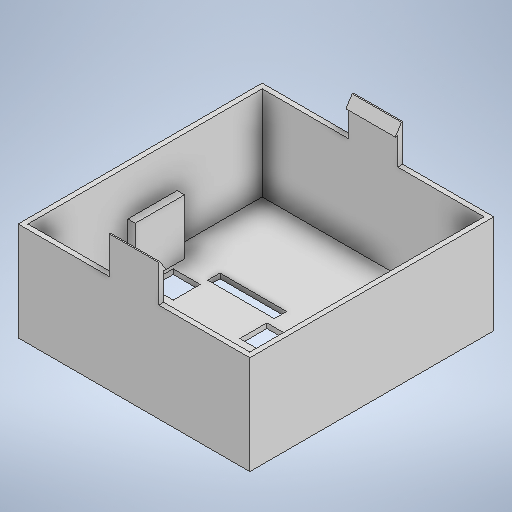
# Autodesk Inventor part: Arduino_case_lid
Saved by Autodesk Inventor 2025.2 (Build 292293000, 293)
## iProperties
Created: 2025-09-19
Part Number: Arduino_case_lid
Material: Generic
Document SubType Name: Modeling
Designer: TSO
Density: 1 g/cm^3
Appearance: Default
Author: TSO
Autodesk Inventor part; units mm, degrees
ref_plane "YZ Plane" through (0, 0, 0) normal (1, 0, 0) x (0, 1, 0)
ref_plane "XZ Plane" through (0, 0, 0) normal (0, 1, 0) x (-1, 0, 0)
ref_plane "XY Plane" through (0, 0, 0) normal (0, 0, 1) x (1, 0, 0)
sketch "Sketch1" plane through (0, 0, 0) normal (0, 1, 0) x (-1, 0, 0)
  line L0 (0, 0) -> (94, 0)
  line L1 (94, 0) -> (94, -99)
  line L2 (94, -99) -> (0, -99)
  line L3 (0, -99) -> (0, 0)
  dimension "d0" = 94
  dimension "d1" = 99
  constraints: 8 end point, 2 parallel, 1 horizontal, 1 perpendicular
  measures "d0" distance of L1.end L2.end
  measures "d1" distance of L0.end L1.end
extrude "Extrusion1" add sketch "Sketch1" along normal blind 40
sketch "Sketch2" plane through (0, 40, 0) normal (0, 1, 0) x (1, 0, 0)
  line L0 (0, 0) -> (0, 99) projected
  line L1 (0, 0) -> (-2, 0)
  line L2 (-2, 0) -> (-2, 2)
  line L3 (-2, 2) -> (0, 2)
  line L4 (0, 2) -> (0, 0)
  line L5 (-2, 2) -> (-92, 2)
  line L6 (-92, 2) -> (-92, 97)
  line L7 (-92, 97) -> (-2, 97)
  line L8 (-2, 97) -> (-2, 2)
  dimension "d4" = 2
  dimension "d5" = 2
  dimension "d6" = 90
  dimension "d7" = 95
  constraints: 16 end point, 4 parallel, 2 horizontal, 2 perpendicular
  measures "d4" distance of L2.end L3.end
  measures "d5" distance of L1.end L2.end
  measures "d6" distance of L6.end L7.end
  measures "d7" distance of L5.end L6.end
extrude "Extrusion2" cut sketch "Sketch2" against normal blind 38 contours L5 L6 L7 L8
sketch "Sketch3" plane through (0, 40, 0) normal (0, 1, 0) x (1, 0, 0)
  line L0 (-92, 97) -> (-2, 97) projected
  line L1 (0, 99) -> (-94, 99) projected
  line L2 (-92, 2) -> (-92, 97) projected
  line L3 (-92, 97) -> (-57, 97)
  line L4 (-92, 97) -> (-57, 97) construction
  line L5 (-57, 97) -> (-37, 97)
  line L6 (-37, 97) -> (-37, 99)
  line L7 (-37, 99) -> (-57, 99)
  line L8 (-57, 99) -> (-57, 97)
  line L9 (-2, 2) -> (-92, 2) projected
  line L10 (-94, 0) -> (0, 0) projected
  line L11 (-57, 2) -> (-37, 2)
  line L12 (-37, 2) -> (-37, 0)
  line L13 (-37, 0) -> (-57, 0)
  line L14 (-57, 0) -> (-57, 2)
  dimension "d11" = 35
  dimension "d12" = 0
  dimension "d13" = 20
  dimension "d14" = 20
  constraints: 20 end point, 4 parallel, 3 horizontal, 3 point on line, 2 collinear, 2 perpendicular
  measures "d11" distance of L0.start L3.end
  measures "d12" distance between parallel lines of L4 L3
  measures "d13" distance of L7.end L6.end
  measures "d14" distance of L12.end L13.end
extrude "Extrusion3" add sketch "Sketch3" along normal blind 15
sketch "Sketch4" plane through (-92, 2, -97) normal (0, 0, 1) x (1, 0, 0)
  line L0 (35, 38) -> (35, 53) projected
  line L1 (35, 53) -> (55, 53)
  line L2 (55, 53) -> (55, 49)
  line L3 (55, 49) -> (35, 49)
  line L4 (35, 49) -> (35, 53)
  point P0 (92, -2)
  dimension "d17" = 20
  dimension "d18" = 4
  constraints: 8 end point, 2 parallel, 1 horizontal, 1 perpendicular
  measures "d17" distance of L2.end L3.end
  measures "d18" distance of L1.end L2.end
extrude "Extrusion4" add sketch "Sketch4" along normal up to surface (95 mm away)
sketch "Sketch5" plane through (0, 55, 0) normal (0, 1, 0) x (1, 0, 0)
  line L0 (-57, 2) -> (-92, 2) projected
  line L1 (-57, 2) -> (-57, 3)
  line L2 (-57, 97) -> (-57, 2) projected
  line L3 (-57, 3) -> (-37, 3)
  line L4 (-37, 3) -> (-37, 96)
  line L5 (-37, 96) -> (-57, 96)
  line L6 (-57, 96) -> (-57, 3)
  point P0 (0, 0)
  dimension "d21" = 1
  dimension "d22" = 93
  constraints: 10 end point, 2 parallel, 1 horizontal, 1 perpendicular, 1 point on line
  measures "d21" distance of L0.start L1.end
  measures "d22" distance of L4.end L3.end
extrude "Extrusion5" cut sketch "Sketch5" against normal up to surface (4 mm away)
chamfer "Chamfer1" distance 2.5 distance2 4 1 edges at (-47, 55, -96) measured on face at (-50.3333, 55, -98)
chamfer "Chamfer2" distance 2.5 distance2 4 1 edges at (-47, 55, -3) measured on face at (-50.3333, 55, -1)
sketch "Sketch6" plane through (0, 2, 0) normal (0, 1, 0) x (1, 0, 0)
  line L0 (-92, 2) -> (-92, 97) projected
  line L1 (-92, 2) -> (-89, 2)
  line L2 (-89, 2) -> (-89, 5) construction
  line L3 (-89, 5) -> (-92, 5) construction
  line L4 (-92, 5) -> (-92, 2)
  line L5 (-89, 5) -> (-89, 39.5) construction
  line L6 (-92, 97) -> (-57, 97) projected
  line L7 (-89, 39.5) -> (-86, 39.5)
  line L8 (-86, 39.5) -> (-86, 59.5)
  line L9 (-86, 59.5) -> (-89, 59.5)
  line L10 (-89, 59.5) -> (-89, 39.5)
  line L11 (0, 99) -> (-94, 99) projected
  line L12 (-47, 99) -> (-47, 0) construction
  line L13 (-94, 0) -> (0, 0) projected
  line L14 (-5, 39.5) -> (-8, 39.5)
  line L15 (-8, 39.5) -> (-8, 59.5)
  line L16 (-8, 59.5) -> (-5, 59.5)
  line L17 (-5, 59.5) -> (-5, 39.5)
  dimension "d31" = 3
  dimension "d32" = 3
  dimension "d33" = 34.5
  dimension "d34" = 3
  dimension "d35" = 20
  dimension "d36" = 37.5
  constraints: 28 end point, 4 parallel, 4 symmetric about line, 3 perpendicular, 2 horizontal, 2 midpoint
  measures "d31" distance of L3.end L2.end
  measures "d32" distance of L2.end L1.end
  measures "d33" distance of L2.end L5.end
  measures "d34" distance of L9.end L8.end
  measures "d35" distance of L8.end L7.end
  measures "d36" distance from line of L6 L9.end
extrude "Extrusion6" add sketch "Sketch6" along normal blind 22.5
sketch "Sketch7" plane through (0, 0, 0) normal (0, -1, 0) x (1, 0, 0)
  line L0 (-94, 0) -> (0, 0) projected
  line L1 (-94, 0) -> (-90, 0)
  line L2 (-90, 0) -> (-90, -4) construction
  line L3 (-90, -4) -> (-94, -4) construction
  line L4 (-94, -4) -> (-94, 0)
  line L5 (-90, -4) -> (-84.8, -4) construction
  line L6 (-84.8, -4) -> (-84.8, -42.7) construction
  line L7 (-84.8, -42.7) -> (-90, -42.7) construction
  line L8 (-90, -42.7) -> (-90, -4) construction
  line L9 (-84.8, -42.7) -> (-73.8, -42.7)
  line L10 (-73.8, -42.7) -> (-73.8, -53.7)
  line L11 (-73.8, -53.7) -> (-84.8, -53.7)
  line L12 (-84.8, -53.7) -> (-84.8, -42.7)
  line L13 (-73.8, -53.7) -> (-46.8, -53.7) construction
  line L14 (-46.8, -53.7) -> (-46.8, -56.7) construction
  line L15 (-46.8, -56.7) -> (-73.8, -56.7) construction
  line L16 (-73.8, -56.7) -> (-73.8, -53.7) construction
  line L17 (-46.8, -56.7) -> (-73.8, -56.7)
  line L18 (-73.8, -56.7) -> (-73.8, -61.7)
  line L19 (-73.8, -61.7) -> (-46.8, -61.7)
  line L20 (-46.8, -61.7) -> (-46.8, -56.7)
  line L21 (-46.8, -53.7) -> (-35.8, -53.7)
  line L22 (-35.8, -53.7) -> (-35.8, -42.7)
  line L23 (-35.8, -42.7) -> (-46.8, -42.7)
  line L24 (-46.8, -42.7) -> (-46.8, -53.7)
  dimension "d39" = 4
  dimension "d40" = 4
  dimension "d41" = 5.2
  dimension "d42" = 38.7
  dimension "d43" = 11
  dimension "d44" = 11
  dimension "d45" = 27
  dimension "d46" = 3
  dimension "d47" = 5
  dimension "d48" = 11
  dimension "d49" = 11
  constraints: 48 end point, 12 parallel, 6 horizontal, 6 perpendicular
  measures "d39" distance of L2.end L3.end
  measures "d40" distance of L1.end L2.end
  measures "d41" distance of L6.end L7.end
  measures "d42" distance of L5.end L6.end
  measures "d43" distance of L10.end L11.end
  measures "d44" distance of L9.end L10.end
  measures "d45" distance of L14.end L15.end
  measures "d46" distance of L13.end L14.end
  measures "d47" distance of L18.end L17.end
  measures "d48" distance of L23.end L22.end
  measures "d49" distance of L22.end L21.end
extrude "Extrusion7" cut sketch "Sketch7" against normal up to surface (2 mm away)
sketch "Sketch8" plane through (0, 0, 0) normal (0, -1, 0) x (1, 0, 0)
  line L0 (0, -99) -> (-94, -99) projected
  line L1 (0, -99) -> (-23.5, -99)
  line L2 (-23.5, -99) -> (-23.5, -89.75)
  line L3 (-23.5, -89.75) -> (0, -89.75)
  line L4 (0, -89.75) -> (0, -99)
  line L5 (-23.5, -89.75) -> (-70.5, -89.75)
  line L6 (-70.5, -89.75) -> (-70.5, -71.25)
  line L7 (-70.5, -71.25) -> (-23.5, -71.25)
  line L8 (-23.5, -71.25) -> (-23.5, -89.75)
  line L9 (-23.3088, -89.836) -> (-70.529, -89.836) construction
  line L10 (-70.529, -89.836) -> (-70.529, -70.9161) construction
  line L11 (-70.529, -70.9161) -> (-23.3088, -70.9161) construction
  line L12 (-23.3088, -70.9161) -> (-23.3088, -89.836) construction
  line L13 (0, -99) -> (-47, -99)
  line L14 (-47, -99) -> (-47, -80.5) construction
  line L15 (-47, -80.5) -> (0, -80.5) construction
  line L16 (0, -80.5) -> (0, -99)
  line L17 (-23.29, -78.926) -> (-24.2676, -81.826)
  line L18 (-24.2676, -81.826) -> (-24.7423, -81.826)
  line L19 (-24.7423, -81.826) -> (-25.72, -78.926)
  line L20 (-25.72, -78.926) -> (-25.3134, -78.926)
  line L21 (-25.3134, -78.926) -> (-25.0502, -79.7368)
  line L22 (-25.0502, -79.7368) -> (-23.9433, -79.7368)
  line L23 (-23.9433, -79.7368) -> (-23.6801, -78.926)
  line L24 (-23.6801, -78.926) -> (-23.29, -78.926)
  line L25 (-24.9444, -80.0658) -> (-24.4956, -81.4312)
  line L26 (-24.4956, -81.4312) -> (-24.0491, -80.0658)
  line L27 (-24.0491, -80.0658) -> (-24.9444, -80.0658)
  line L28 (-27.0055, -78.926) -> (-25.8821, -78.926)
  line L29 (-25.8821, -78.926) -> (-25.8821, -79.2222)
  line L30 (-25.8821, -79.2222) -> (-26.2511, -79.2222)
  line L31 (-26.2511, -79.2222) -> (-26.2511, -81.5299)
  line L32 (-26.2511, -81.5299) -> (-25.8821, -81.5299)
  line L33 (-25.8821, -81.5299) -> (-25.8821, -81.826)
  line L34 (-25.8821, -81.826) -> (-27.0055, -81.826)
  line L35 (-27.0055, -81.826) -> (-27.0055, -81.5299)
  line L36 (-27.0055, -81.5299) -> (-26.6365, -81.5299)
  line L37 (-26.6365, -81.5299) -> (-26.6365, -79.2222)
  line L38 (-26.6365, -79.2222) -> (-27.0055, -79.2222)
  line L39 (-27.0055, -79.2222) -> (-27.0055, -78.926)
  line L40 (-29.7269, -78.926) -> (-29.2263, -78.926)
  line L41 (-29.2263, -78.926) -> (-28.3098, -80.0799)
  line L42 (-28.3098, -80.0799) -> (-27.8679, -80.0799)
  line L43 (-27.8679, -80.0799) -> (-27.8679, -78.926)
  line L44 (-27.8679, -78.926) -> (-27.4825, -78.926)
  line L45 (-27.4825, -78.926) -> (-27.4825, -81.826)
  line L46 (-27.4825, -81.826) -> (-28.2299, -81.826)
  spline S0 degree 2 poles (-28.2299, -81.826) (-28.479, -81.826) (-28.815, -81.772) (-28.9678, -81.6733) knots 0 0 0 1 2 2 2
  spline S1 degree 2 poles (-28.9678, -81.6733) (-29.1205, -81.5746) (-29.2968, -81.2667) (-29.2968, -81.0388) knots 0 0 0 1 2 2 2
  spline S2 degree 2 poles (-29.2968, -81.0388) (-29.2968, -80.7215) (-28.9725, -80.2914) (-28.6952, -80.188) knots 0 0 0 1 2 2 2
  line L47 (-28.6952, -80.188) -> (-29.7269, -78.926)
  spline S3 degree 2 poles (-28.8949, -81.0082) (-28.8949, -81.1351) (-28.8056, -81.3302) (-28.7116, -81.3936) knots 0 0 0 1 2 2 2
  spline S4 degree 2 poles (-28.7116, -81.3936) (-28.6294, -81.4477) (-28.4108, -81.4923) (-28.251, -81.4923) knots 0 0 0 1 2 2 2
  line L48 (-28.251, -81.4923) -> (-27.8679, -81.4923)
  line L49 (-27.8679, -81.4923) -> (-27.8679, -80.4019)
  line L50 (-27.8679, -80.4019) -> (-28.2064, -80.4019)
  spline S5 degree 2 poles (-28.2064, -80.4019) (-28.3732, -80.4019) (-28.6388, -80.4606) (-28.7304, -80.5523) knots 0 0 0 1 2 2 2
  spline S6 degree 2 poles (-28.7304, -80.5523) (-28.815, -80.6322) (-28.8949, -80.8578) (-28.8949, -81.0082) knots 0 0 0 1 2 2 2
  line L51 (-33.3084, -78.926) -> (-32.923, -78.926)
  line L52 (-32.923, -78.926) -> (-32.923, -80.3455)
  line L53 (-32.923, -80.3455) -> (-31.5881, -80.3455)
  line L54 (-31.5881, -80.3455) -> (-31.5881, -78.926)
  line L55 (-31.5881, -78.926) -> (-31.2027, -78.926)
  line L56 (-31.2027, -78.926) -> (-31.2027, -81.826)
  line L57 (-31.2027, -81.826) -> (-31.5881, -81.826)
  line L58 (-31.5881, -81.826) -> (-31.5881, -80.6886)
  line L59 (-31.5881, -80.6886) -> (-32.923, -80.6886)
  line L60 (-32.923, -80.6886) -> (-32.923, -81.826)
  line L61 (-32.923, -81.826) -> (-33.3084, -81.826)
  line L62 (-33.3084, -81.826) -> (-33.3084, -78.926)
  line L63 (-33.8959, -78.926) -> (-33.8959, -81.826)
  line L64 (-33.8959, -81.826) -> (-35.7102, -81.826)
  line L65 (-35.7102, -81.826) -> (-35.7102, -81.4829)
  line L66 (-35.7102, -81.4829) -> (-34.2813, -81.4829)
  line L67 (-34.2813, -81.4829) -> (-34.2813, -80.6886)
  line L68 (-34.2813, -80.6886) -> (-35.6138, -80.6886)
  line L69 (-35.6138, -80.6886) -> (-35.6138, -80.3455)
  line L70 (-35.6138, -80.3455) -> (-34.2813, -80.3455)
  line L71 (-34.2813, -80.3455) -> (-34.2813, -79.2692)
  line L72 (-34.2813, -79.2692) -> (-35.7102, -79.2692)
  line L73 (-35.7102, -79.2692) -> (-35.7102, -78.926)
  line L74 (-35.7102, -78.926) -> (-33.8959, -78.926)
  line L75 (-35.8206, -78.926) -> (-36.7983, -81.826)
  line L76 (-36.7983, -81.826) -> (-37.273, -81.826)
  line L77 (-37.273, -81.826) -> (-38.2506, -78.926)
  line L78 (-38.2506, -78.926) -> (-37.844, -78.926)
  line L79 (-37.844, -78.926) -> (-37.5808, -79.7368)
  line L80 (-37.5808, -79.7368) -> (-36.4739, -79.7368)
  line L81 (-36.4739, -79.7368) -> (-36.2107, -78.926)
  line L82 (-36.2107, -78.926) -> (-35.8206, -78.926)
  line L83 (-37.4751, -80.0658) -> (-37.0262, -81.4312)
  line L84 (-37.0262, -81.4312) -> (-36.5797, -80.0658)
  line L85 (-36.5797, -80.0658) -> (-37.4751, -80.0658)
  line L86 (-39.2024, -78.926) -> (-39.2024, -81.4829)
  line L87 (-39.2024, -81.4829) -> (-38.2295, -81.4829)
  line L88 (-38.2295, -81.4829) -> (-38.2295, -81.826)
  line L89 (-38.2295, -81.826) -> (-40.5607, -81.826)
  line L90 (-40.5607, -81.826) -> (-40.5607, -81.4829)
  line L91 (-40.5607, -81.4829) -> (-39.5878, -81.4829)
  line L92 (-39.5878, -81.4829) -> (-39.5878, -78.926)
  line L93 (-39.5878, -78.926) -> (-39.2024, -78.926)
  line L94 (-40.8545, -78.926) -> (-40.8545, -81.826)
  line L95 (-40.8545, -81.826) -> (-42.6688, -81.826)
  line L96 (-42.6688, -81.826) -> (-42.6688, -81.4829)
  line L97 (-42.6688, -81.4829) -> (-41.2399, -81.4829)
  line L98 (-41.2399, -81.4829) -> (-41.2399, -80.6886)
  line L99 (-41.2399, -80.6886) -> (-42.5724, -80.6886)
  line L100 (-42.5724, -80.6886) -> (-42.5724, -80.3455)
  line L101 (-42.5724, -80.3455) -> (-41.2399, -80.3455)
  line L102 (-41.2399, -80.3455) -> (-41.2399, -79.2692)
  line L103 (-41.2399, -79.2692) -> (-42.6688, -79.2692)
  line L104 (-42.6688, -79.2692) -> (-42.6688, -78.926)
  line L105 (-42.6688, -78.926) -> (-40.8545, -78.926)
  line L106 (-45.3361, -78.926) -> (-44.8355, -78.926)
  line L107 (-44.8355, -78.926) -> (-43.919, -80.0799)
  line L108 (-43.919, -80.0799) -> (-43.4772, -80.0799)
  line L109 (-43.4772, -80.0799) -> (-43.4772, -78.926)
  line L110 (-43.4772, -78.926) -> (-43.0918, -78.926)
  line L111 (-43.0918, -78.926) -> (-43.0918, -81.826)
  line L112 (-43.0918, -81.826) -> (-43.8391, -81.826)
  spline S7 degree 2 poles (-43.8391, -81.826) (-44.0882, -81.826) (-44.4243, -81.772) (-44.577, -81.6733) knots 0 0 0 1 2 2 2
  spline S8 degree 2 poles (-44.577, -81.6733) (-44.7298, -81.5746) (-44.906, -81.2667) (-44.906, -81.0388) knots 0 0 0 1 2 2 2
  spline S9 degree 2 poles (-44.906, -81.0388) (-44.906, -80.7215) (-44.5817, -80.2914) (-44.3044, -80.188) knots 0 0 0 1 2 2 2
  line L113 (-44.3044, -80.188) -> (-45.3361, -78.926)
  spline S10 degree 2 poles (-44.5042, -81.0082) (-44.5042, -81.1351) (-44.4149, -81.3302) (-44.3209, -81.3936) knots 0 0 0 1 2 2 2
  spline S11 degree 2 poles (-44.3209, -81.3936) (-44.2386, -81.4477) (-44.0201, -81.4923) (-43.8602, -81.4923) knots 0 0 0 1 2 2 2
  line L114 (-43.8602, -81.4923) -> (-43.4772, -81.4923)
  line L115 (-43.4772, -81.4923) -> (-43.4772, -80.4019)
  line L116 (-43.4772, -80.4019) -> (-43.8156, -80.4019)
  spline S12 degree 2 poles (-43.8156, -80.4019) (-43.9825, -80.4019) (-44.248, -80.4606) (-44.3397, -80.5523) knots 0 0 0 1 2 2 2
  spline S13 degree 2 poles (-44.3397, -80.5523) (-44.4243, -80.6322) (-44.5042, -80.8578) (-44.5042, -81.0082) knots 0 0 0 1 2 2 2
  spline S14 degree 2 poles (-47.9447, -78.8743) (-47.6627, -78.8743) (-47.1856, -79.0647) (-47.0117, -79.2551) knots 0 0 0 1 2 2 2
  spline S15 degree 2 poles (-47.0117, -79.2551) (-46.8378, -79.4431) (-46.6474, -80.0071) (-46.6474, -80.3737) knots 0 0 0 1 2 2 2
  spline S16 degree 2 poles (-46.6474, -80.3737) (-46.6474, -80.738) (-46.8331, -81.2785) (-47.0094, -81.4782) knots 0 0 0 1 2 2 2
  spline S17 degree 2 poles (-47.0094, -81.4782) (-47.1833, -81.6733) (-47.658, -81.8777) (-47.9517, -81.8777) knots 0 0 0 1 2 2 2
  spline S18 degree 2 poles (-47.9517, -81.8777) (-48.0974, -81.8777) (-48.3536, -81.8354) (-48.4617, -81.8025) knots 0 0 0 1 2 2 2
  spline S19 degree 2 poles (-48.4617, -81.8025) (-48.5557, -81.772) (-48.7508, -81.685) (-48.8471, -81.6333) knots 0 0 0 1 2 2 2
  line L117 (-48.8471, -81.6333) -> (-48.8471, -81.168)
  line L118 (-48.8471, -81.168) -> (-48.8166, -81.168)
  spline S20 degree 2 poles (-48.8166, -81.168) (-48.7649, -81.215) (-48.6051, -81.3466) (-48.4899, -81.4101) knots 0 0 0 1 2 2 2
  spline S21 degree 2 poles (-48.4899, -81.4101) (-48.3795, -81.4712) (-48.1186, -81.5487) (-47.9494, -81.5487) knots 0 0 0 1 2 2 2
  spline S22 degree 2 poles (-47.9494, -81.5487) (-47.7637, -81.5487) (-47.4324, -81.396) (-47.3078, -81.2503) knots 0 0 0 1 2 2 2
  spline S23 degree 2 poles (-47.3078, -81.2503) (-47.1856, -81.1022) (-47.0493, -80.6534) (-47.0493, -80.3737) knots 0 0 0 1 2 2 2
  spline S24 degree 2 poles (-47.0493, -80.3737) (-47.0493, -80.0752) (-47.1927, -79.6452) (-47.3172, -79.4971) knots 0 0 0 1 2 2 2
  spline S25 degree 2 poles (-47.3172, -79.4971) (-47.4394, -79.3538) (-47.7661, -79.2081) (-47.9494, -79.2081) knots 0 0 0 1 2 2 2
  spline S26 degree 2 poles (-47.9494, -79.2081) (-48.1162, -79.2081) (-48.4006, -79.2903) (-48.5111, -79.3514) knots 0 0 0 1 2 2 2
  spline S27 degree 2 poles (-48.5111, -79.3514) (-48.6168, -79.4125) (-48.7743, -79.5394) (-48.8189, -79.5841) knots 0 0 0 1 2 2 2
  line L119 (-48.8189, -79.5841) -> (-48.8471, -79.5841)
  line L120 (-48.8471, -79.5841) -> (-48.8471, -79.1235)
  spline S28 degree 2 poles (-48.8471, -79.1235) (-48.7508, -79.0788) (-48.5816, -78.9965) (-48.4617, -78.9589) knots 0 0 0 1 2 2 2
  spline S29 degree 2 poles (-48.4617, -78.9589) (-48.3348, -78.9166) (-48.1186, -78.8743) (-47.9447, -78.8743) knots 0 0 0 1 2 2 2
  spline S30 degree 2 poles (-51.2583, -81.4947) (-51.4228, -81.302) (-51.6061, -80.738) (-51.6061, -80.376) knots 0 0 0 1 2 2 2
  spline S31 degree 2 poles (-51.6061, -80.376) (-51.6061, -80.0235) (-51.4275, -79.4525) (-51.2583, -79.2598) knots 0 0 0 1 2 2 2
  spline S32 degree 2 poles (-51.2583, -79.2598) (-51.0797, -79.0577) (-50.6073, -78.8649) (-50.323, -78.8649) knots 0 0 0 1 2 2 2
  spline S33 degree 2 poles (-50.323, -78.8649) (-50.0292, -78.8649) (-49.5592, -79.0647) (-49.3876, -79.2598) knots 0 0 0 1 2 2 2
  spline S34 degree 2 poles (-49.3876, -79.2598) (-49.2208, -79.4525) (-49.0422, -80.0188) (-49.0422, -80.376) knots 0 0 0 1 2 2 2
  spline S35 degree 2 poles (-49.0422, -80.376) (-49.0422, -80.7403) (-49.2231, -81.2949) (-49.39, -81.4947) knots 0 0 0 1 2 2 2
  spline S36 degree 2 poles (-49.39, -81.4947) (-49.5592, -81.6874) (-50.0316, -81.8871) (-50.323, -81.8871) knots 0 0 0 1 2 2 2
  spline S37 degree 2 poles (-50.323, -81.8871) (-50.6191, -81.8871) (-51.0938, -81.6803) (-51.2583, -81.4947) knots 0 0 0 1 2 2 2
  spline S38 degree 2 poles (-51.2043, -80.376) (-51.2043, -80.6628) (-51.0797, -81.1069) (-50.9669, -81.2526) knots 0 0 0 1 2 2 2
  spline S39 degree 2 poles (-50.9669, -81.2526) (-50.8517, -81.403) (-50.5274, -81.5534) (-50.3253, -81.5534) knots 0 0 0 1 2 2 2
  spline S40 degree 2 poles (-50.3253, -81.5534) (-50.1162, -81.5534) (-49.8013, -81.4077) (-49.6814, -81.2526) knots 0 0 0 1 2 2 2
  spline S41 degree 2 poles (-49.6814, -81.2526) (-49.5662, -81.1046) (-49.444, -80.6581) (-49.444, -80.376) knots 0 0 0 1 2 2 2
  spline S42 degree 2 poles (-49.444, -80.376) (-49.444, -79.805) (-49.9235, -79.1987) (-50.3253, -79.1987) knots 0 0 0 1 2 2 2
  spline S43 degree 2 poles (-50.3253, -79.1987) (-50.7272, -79.1987) (-51.2043, -79.805) (-51.2043, -80.376) knots 0 0 0 1 2 2 2
  line L121 (-54.1043, -78.926) -> (-53.6718, -78.926)
  line L122 (-53.6718, -78.926) -> (-52.3887, -81.4265)
  line L123 (-52.3887, -81.4265) -> (-52.3887, -78.926)
  line L124 (-52.3887, -78.926) -> (-52.0291, -78.926)
  line L125 (-52.0291, -78.926) -> (-52.0291, -81.826)
  line L126 (-52.0291, -81.826) -> (-52.5767, -81.826)
  line L127 (-52.5767, -81.826) -> (-53.7447, -79.53)
  line L128 (-53.7447, -79.53) -> (-53.7447, -81.826)
  line L129 (-53.7447, -81.826) -> (-54.1043, -81.826)
  line L130 (-54.1043, -81.826) -> (-54.1043, -78.926)
  line L131 (-55.3686, -78.926) -> (-55.3686, -81.4829)
  line L132 (-55.3686, -81.4829) -> (-54.3957, -81.4829)
  line L133 (-54.3957, -81.4829) -> (-54.3957, -81.826)
  line L134 (-54.3957, -81.826) -> (-56.7269, -81.826)
  line L135 (-56.7269, -81.826) -> (-56.7269, -81.4829)
  line L136 (-56.7269, -81.4829) -> (-55.754, -81.4829)
  line L137 (-55.754, -81.4829) -> (-55.754, -78.926)
  line L138 (-55.754, -78.926) -> (-55.3686, -78.926)
  line L139 (-59.265, -78.926) -> (-58.7645, -78.926)
  line L140 (-58.7645, -78.926) -> (-57.8479, -80.0799)
  line L141 (-57.8479, -80.0799) -> (-57.4061, -80.0799)
  line L142 (-57.4061, -80.0799) -> (-57.4061, -78.926)
  line L143 (-57.4061, -78.926) -> (-57.0207, -78.926)
  line L144 (-57.0207, -78.926) -> (-57.0207, -81.826)
  line L145 (-57.0207, -81.826) -> (-57.768, -81.826)
  spline S44 degree 2 poles (-57.768, -81.826) (-58.0171, -81.826) (-58.3532, -81.772) (-58.506, -81.6733) knots 0 0 0 1 2 2 2
  spline S45 degree 2 poles (-58.506, -81.6733) (-58.6587, -81.5746) (-58.835, -81.2667) (-58.835, -81.0388) knots 0 0 0 1 2 2 2
  spline S46 degree 2 poles (-58.835, -81.0388) (-58.835, -80.7215) (-58.5107, -80.2914) (-58.2333, -80.188) knots 0 0 0 1 2 2 2
  line L146 (-58.2333, -80.188) -> (-59.265, -78.926)
  spline S47 degree 2 poles (-58.4331, -81.0082) (-58.4331, -81.1351) (-58.3438, -81.3302) (-58.2498, -81.3936) knots 0 0 0 1 2 2 2
  spline S48 degree 2 poles (-58.2498, -81.3936) (-58.1675, -81.4477) (-57.949, -81.4923) (-57.7892, -81.4923) knots 0 0 0 1 2 2 2
  line L147 (-57.7892, -81.4923) -> (-57.4061, -81.4923)
  line L148 (-57.4061, -81.4923) -> (-57.4061, -80.4019)
  line L149 (-57.4061, -80.4019) -> (-57.7445, -80.4019)
  spline S49 degree 2 poles (-57.7445, -80.4019) (-57.9114, -80.4019) (-58.1769, -80.4606) (-58.2686, -80.5523) knots 0 0 0 1 2 2 2
  spline S50 degree 2 poles (-58.2686, -80.5523) (-58.3532, -80.6322) (-58.4331, -80.8578) (-58.4331, -81.0082) knots 0 0 0 1 2 2 2
  spline S51 degree 2 poles (-61.547, -81.4947) (-61.7115, -81.302) (-61.8948, -80.738) (-61.8948, -80.376) knots 0 0 0 1 2 2 2
  spline S52 degree 2 poles (-61.8948, -80.376) (-61.8948, -80.0235) (-61.7162, -79.4525) (-61.547, -79.2598) knots 0 0 0 1 2 2 2
  spline S53 degree 2 poles (-61.547, -79.2598) (-61.3684, -79.0577) (-60.896, -78.8649) (-60.6116, -78.8649) knots 0 0 0 1 2 2 2
  spline S54 degree 2 poles (-60.6116, -78.8649) (-60.3179, -78.8649) (-59.8479, -79.0647) (-59.6763, -79.2598) knots 0 0 0 1 2 2 2
  spline S55 degree 2 poles (-59.6763, -79.2598) (-59.5094, -79.4525) (-59.3308, -80.0188) (-59.3308, -80.376) knots 0 0 0 1 2 2 2
  spline S56 degree 2 poles (-59.3308, -80.376) (-59.3308, -80.7403) (-59.5118, -81.2949) (-59.6786, -81.4947) knots 0 0 0 1 2 2 2
  spline S57 degree 2 poles (-59.6786, -81.4947) (-59.8479, -81.6874) (-60.3202, -81.8871) (-60.6116, -81.8871) knots 0 0 0 1 2 2 2
  spline S58 degree 2 poles (-60.6116, -81.8871) (-60.9077, -81.8871) (-61.3825, -81.6803) (-61.547, -81.4947) knots 0 0 0 1 2 2 2
  spline S59 degree 2 poles (-61.4929, -80.376) (-61.4929, -80.6628) (-61.3684, -81.1069) (-61.2555, -81.2526) knots 0 0 0 1 2 2 2
  spline S60 degree 2 poles (-61.2555, -81.2526) (-61.1404, -81.403) (-60.8161, -81.5534) (-60.614, -81.5534) knots 0 0 0 1 2 2 2
  spline S61 degree 2 poles (-60.614, -81.5534) (-60.4048, -81.5534) (-60.0899, -81.4077) (-59.9701, -81.2526) knots 0 0 0 1 2 2 2
  spline S62 degree 2 poles (-59.9701, -81.2526) (-59.8549, -81.1046) (-59.7327, -80.6581) (-59.7327, -80.376) knots 0 0 0 1 2 2 2
  spline S63 degree 2 poles (-59.7327, -80.376) (-59.7327, -79.805) (-60.2121, -79.1987) (-60.614, -79.1987) knots 0 0 0 1 2 2 2
  spline S64 degree 2 poles (-60.614, -79.1987) (-61.0158, -79.1987) (-61.4929, -79.805) (-61.4929, -80.376) knots 0 0 0 1 2 2 2
  line L150 (-63.9981, -78.926) -> (-62.3178, -78.926)
  line L151 (-62.3178, -78.926) -> (-62.3178, -81.826)
  line L152 (-62.3178, -81.826) -> (-62.7032, -81.826)
  line L153 (-62.7032, -81.826) -> (-62.7032, -79.2692)
  line L154 (-62.7032, -79.2692) -> (-63.9981, -79.2692)
  line L155 (-63.9981, -79.2692) -> (-63.9981, -78.926)
  line L156 (-65.9816, -78.926) -> (-64.3013, -78.926)
  line L157 (-64.3013, -78.926) -> (-64.3013, -81.826)
  line L158 (-64.3013, -81.826) -> (-64.6867, -81.826)
  line L159 (-64.6867, -81.826) -> (-64.6867, -79.2692)
  line L160 (-64.6867, -79.2692) -> (-65.9816, -79.2692)
  line L161 (-65.9816, -79.2692) -> (-65.9816, -78.926)
  line L162 (-66.2847, -78.926) -> (-66.2847, -81.826)
  line L163 (-66.2847, -81.826) -> (-68.099, -81.826)
  line L164 (-68.099, -81.826) -> (-68.099, -81.4829)
  line L165 (-68.099, -81.4829) -> (-66.6701, -81.4829)
  line L166 (-66.6701, -81.4829) -> (-66.6701, -80.6886)
  line L167 (-66.6701, -80.6886) -> (-68.0026, -80.6886)
  line L168 (-68.0026, -80.6886) -> (-68.0026, -80.3455)
  line L169 (-68.0026, -80.3455) -> (-66.6701, -80.3455)
  line L170 (-66.6701, -80.3455) -> (-66.6701, -79.2692)
  line L171 (-66.6701, -79.2692) -> (-68.099, -79.2692)
  line L172 (-68.099, -79.2692) -> (-68.099, -78.926)
  line L173 (-68.099, -78.926) -> (-66.2847, -78.926)
  line L174 (-70.7663, -78.926) -> (-70.2658, -78.926)
  line L175 (-70.2658, -78.926) -> (-69.3492, -80.0799)
  line L176 (-69.3492, -80.0799) -> (-68.9074, -80.0799)
  line L177 (-68.9074, -80.0799) -> (-68.9074, -78.926)
  line L178 (-68.9074, -78.926) -> (-68.522, -78.926)
  line L179 (-68.522, -78.926) -> (-68.522, -81.826)
  line L180 (-68.522, -81.826) -> (-69.2693, -81.826)
  spline S65 degree 2 poles (-69.2693, -81.826) (-69.5184, -81.826) (-69.8545, -81.772) (-70.0073, -81.6733) knots 0 0 0 1 2 2 2
  spline S66 degree 2 poles (-70.0073, -81.6733) (-70.16, -81.5746) (-70.3363, -81.2667) (-70.3363, -81.0388) knots 0 0 0 1 2 2 2
  spline S67 degree 2 poles (-70.3363, -81.0388) (-70.3363, -80.7215) (-70.012, -80.2914) (-69.7346, -80.188) knots 0 0 0 1 2 2 2
  line L181 (-69.7346, -80.188) -> (-70.7663, -78.926)
  spline S68 degree 2 poles (-69.9344, -81.0082) (-69.9344, -81.1351) (-69.8451, -81.3302) (-69.7511, -81.3936) knots 0 0 0 1 2 2 2
  spline S69 degree 2 poles (-69.7511, -81.3936) (-69.6688, -81.4477) (-69.4503, -81.4923) (-69.2905, -81.4923) knots 0 0 0 1 2 2 2
  line L182 (-69.2905, -81.4923) -> (-68.9074, -81.4923)
  line L183 (-68.9074, -81.4923) -> (-68.9074, -80.4019)
  line L184 (-68.9074, -80.4019) -> (-69.2458, -80.4019)
  spline S70 degree 2 poles (-69.2458, -80.4019) (-69.4127, -80.4019) (-69.6782, -80.4606) (-69.7699, -80.5523) knots 0 0 0 1 2 2 2
  spline S71 degree 2 poles (-69.7699, -80.5523) (-69.8545, -80.6322) (-69.9344, -80.8578) (-69.9344, -81.0082) knots 0 0 0 1 2 2 2
  point P0 (0, 0)
  dimension "d52" = 23.5
  dimension "d53" = 9.25
  dimension "d54" = 47
  dimension "d55" = 18.5
  dimension "d56" = 47
  dimension "d57" = 18.5
  constraints: 24 end point, 6 parallel, 3 horizontal, 3 perpendicular, 2 other
  measures "d52" distance of L2.end L3.end
  measures "d53" distance of L1.end L2.end
  measures "d54" distance of L6.end L7.end
  measures "d55" distance of L5.end L6.end
  measures "d56" distance of L14.end L15.end
  measures "d57" distance of L13.end L14.end
extrude "Extrusion8" cut sketch "Sketch8" against normal blind 0.2 contours L17 L18 L19 L20 L21 L22 L23 L24 L8 | L8 L24 L17 | L181 L174 L6 | L6 L174 L175 L176 L177 L178 L179 L180 S65 S66 S67 L181 | L28 L29 L30 L31 L32 L33 L34 L35 L36 L37 L38 L39 | L40 L41 L42 L43 L44 L45 L46 S0 S1 S2 L47 | L51 L52 L53 L54 L55 L56 L57 L58 L59 L60 L61 L62 | L63 L64 L65 L66 L67 L68 L69 L70 L71 L72 L73 L74 | L75 L76 L77 L78 L79 L80 L81 L82 | L86 L87 L88 L89 L90 L91 L92 L93 | L94 L95 L96 L97 L98 L99 L100 L101 L102 L103 L104 L105 | L106 L107 L108 L109 L110 L111 L112 S7 S8 S9 L113 | S14 S15 S16 S17 S18 S19 L117 L118 S20 S21 S22 S23 S24 S25 S26 S27 L119 L120 S28 S29 | S30 S31 S32 S33 S34 S35 S36 S37 | L121 L122 L123 L124 L125 L126 L127 L128 L129 L130 | L131 L132 L133 L134 L135 L136 L137 L138 | L139 L140 L141 L142 L143 L144 L145 S44 S45 S46 L146 | S51 S52 S53 S54 S55 S56 S57 S58 | L150 L151 L152 L153 L154 L155 | L156 L157 L158 L159 L160 L161 | L162 L163 L164 L165 L166 L167 L168 L169 L170 L171 L172 L173
body "Solid1"
